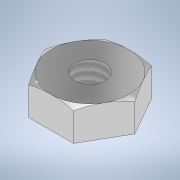
# Autodesk Inventor part: M3-HexaNut-type2
Saved by Autodesk Inventor 2022.2 (Build 262287000, 287)
## iProperties
Created: 2022-02-28
Part Number: M3-HexaNut-type2
Material: 一般
Document SubType Name: Modeling
Designer: Yuta Fujiyama
Density: 1 g/cm^3
Appearance: クローム - つや出し
Author: Yuta Fujiyama
Autodesk Inventor part; units mm, degrees
ref_plane "YZ Plane" through (0, 0, 0) normal (1, 0, 0) x (0, 1, 0)
ref_plane "XZ Plane" through (0, 0, 0) normal (0, 1, 0) x (-1, 0, 0)
ref_plane "XY Plane" through (0, 0, 0) normal (0, 0, 1) x (1, 0, 0)
sketch "スケッチ1" plane through (0, 0, 0) normal (0, 1, 0) x (-1, 0, 0)
  circle A0 centre (0, 0) radius 2.3094 construction
  line L0 (2.3094, 0) -> (1.1547, 2)
  line L1 (1.1547, 2) -> (-1.1547, 2)
  line L2 (-1.1547, 2) -> (-2.3094, 0)
  line L3 (-2.3094, 0) -> (-1.1547, -2)
  line L4 (-1.1547, -2) -> (1.1547, -2)
  line L5 (1.1547, -2) -> (2.3094, 0)
  dimension "d0" = 4
  constraints: 12 end point, 6 point on circle, 4 equal length, 2 horizontal, 1 centre point, 1 coincident
  measures "d0" distance between parallel lines of L4 L1
extrude "押し出し1" add sketch "スケッチ1" along normal blind 1.6
sketch "スケッチ2" plane through (0, 1.6, 0) normal (0, 1, 0) x (1, 0, 0)
  point P0 (0, 0)
  point P1 (0, 0)
  constraints: 1 coincident
hole "穴1" at (0, 1.6, 0) direction (0, -1, 0) diameter 1.567 end through all thread size "M2x0.4" class "6H" standard "ISO Metric profile"
sketch "スケッチ3" plane through (0, 0, 0) normal (1, 0, 0) x (0, 1, 0)
  arc A0 (1.0174, -3) -> (1.6, -2) centre (-2.9826, 0) ccw
  line L0 (0, -2) -> (1.6, -2) construction
  line L1 (1.6, -3) -> (1.0174, -3)
  line L2 (1.6, 0.7835) -> (1.6, -0.7835) construction
  line L3 (1.6, -2) -> (1.6, -3)
  line L4 (-3.9049, 0) -> (2.5514, 0) projected
  point P0 (0, 0)
  point P1 (1.6, 0)
  dimension "d10" = 2
  dimension "d11" = 5
  dimension "d12" = 1
  constraints: 4 end point, 2 point on circle, 1 centre point, 1 collinear, 1 horizontal alignment, 1 midpoint, 1 perpendicular
  measures "d10" distance of L3.start point (1.6, 0)
  measures "d11" radius of A0
  measures "d12" distance of L3.start L1.start
revolve "回転1" cut sketch "スケッチ3" angle 360 about axis through (0, -10, 0) along (0, 1, 0)
